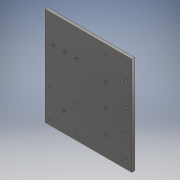
# Autodesk Inventor part: HeadPlate
Saved by Autodesk Inventor 2017 (Build 210142000, 142)
## iProperties
Created: 2016-12-13
Part Number: HeadPlate
Material: Steel, Carbon
Document SubType Name: Modeling
Designer: umr
Density: 7.85 g/cm^3
Appearance: Semi-Polished
Mass: 989.197 g
Surface Area: 546.459 cm^2
Volume: 126.012 cm^3
Author: umr
Autodesk Inventor part; units mm, degrees
ref_plane "YZ Plane" through (0, 0, 0) normal (1, 0, 0) x (0, 1, 0)
ref_plane "XZ Plane" through (0, 0, 0) normal (0, 1, 0) x (-1, 0, 0)
ref_plane "XY Plane" through (0, 0, 0) normal (0, 0, 1) x (1, 0, 0)
sketch "Sketch1" plane through (0, 0, 0) normal (0, 1, 0) x (-1, 0, 0)
  line L0 (0, 0) -> (150, 0)
  line L1 (150, 0) -> (150, -170)
  line L2 (150, -170) -> (0, -170)
  line L3 (0, -170) -> (0, 0)
  dimension "d0" = 150
  dimension "d1" = 170
  constraints: 8 end point, 2 parallel, 1 horizontal, 1 perpendicular
  measures "d0" distance of L1.end L2.end
  measures "d1" distance of L0.end L1.end
extrude "Extrusion1" add sketch "Sketch1" along normal blind 5
sketch "Sketch2" plane through (0, 5, 0) normal (0, 1, 0) x (1, 0, 0)
  line L0 (-150, 170) -> (-150, 0) projected
  line L1 (-150, 0) -> (0, 0) projected
  line L2 (0, 0) -> (0, 170) projected
  line L3 (0, 170) -> (-150, 170) projected
  circle A0 centre (-117, 137) radius 2.75
  circle A1 centre (-140.5, 160.5) radius 1.75
  circle A2 centre (-140.5, 113.5) radius 1.75
  circle A3 centre (-93.5, 160.5) radius 1.75
  circle A4 centre (-93.5, 113.5) radius 1.75
  circle A5 centre (-45, 137) radius 2.75
  circle A6 centre (-10, 157) radius 2.75
  circle A7 centre (-115, 47.5) radius 2.75
  circle A8 centre (-95, 47.5) radius 2.75
  circle A9 centre (-135, 47.5) radius 2.75
  circle A10 centre (-45, 97) radius 2.75
  circle A11 centre (-45, 57) radius 2.75
  circle A12 centre (-45, 17) radius 2.75
  circle A13 centre (-10, 117) radius 2.75
  circle A14 centre (-10, 77) radius 2.75
  circle A15 centre (-10, 37) radius 2.75
  dimension "d5" = 5.5
  dimension "d8" = 3.5
  dimension "d9" = 9.5
  dimension "d10" = 9.5
  dimension "d13" = 47
  dimension "d16" = 47
  dimension "d23" = 5.5
  dimension "d24" = 5.5
  dimension "d25" = 33
  dimension "d26" = 13
  dimension "d28" = 170
  dimension "d36" = 10
  dimension "d40" = 45
  dimension "d43" = 5.5
  dimension "d44" = 5.5
  dimension "d48" = 20
  dimension "d49" = 35
  dimension "d50" = 5.5
  dimension "d51" = 20
  dimension "d53" = 23.5
  dimension "d54" = 23.5
  dimension "d55" = 33
  dimension "d58" = 40
  dimension "d65" = 40
  constraints: 16 centre point, 3 vertical, 1 horizontal, 18 other
  measures "d5" diameter of A0
  measures "d8" diameter of A1
  measures "d9" distance from line of A1.centre L3
  measures "d10" distance from line of L0 A1.centre
  measures "d13" distance of A1.centre A2.centre
  measures "d16" distance of A1.centre A3.centre
  measures "d23" diameter of A5
  measures "d24" diameter of A6
  measures "d25" distance from line of L3 A5.centre
  measures "d26" distance from line of L3 A6.centre
  measures "d28" distance between parallel lines of L3 L1
  measures "d36" distance from line of L2 A6.centre
  measures "d40" distance from line of L2 A5.centre
  measures "d43" diameter of A7
  measures "d44" diameter of A8
  measures "d48" distance of A7.centre A8.centre
  measures "d49" distance from line of L0 A7.centre
  measures "d50" diameter of A9
  measures "d51" distance of A9.centre A7.centre
  measures "d53" horizontal distance of A0.centre A1.centre
  measures "d54" horizontal distance of A4.centre A0.centre
  measures "d55" distance from line of L3 A0.centre
  measures "d58" distance of A5.centre A10.centre
  measures "d65" distance of A6.centre A13.centre
extrude "Extrusion3" cut sketch "Sketch2" against normal blind 10 contours A0 | A1 | A2 | A3 | A4 | A5 | A6 | A7 | A8 | A9 | A10 | A11 | A12 | A13 | A14 | A15
equation "\"d16\" = d13"
equation "\"d36\" = d34"
equation "\"d40\" = d37"
equation "\"d53\" = 0.5 * d13"
equation "\"d54\" = d53"
equation "\"d34\" = 10"
equation "\"d37\" = 45"
body "Solid1"
